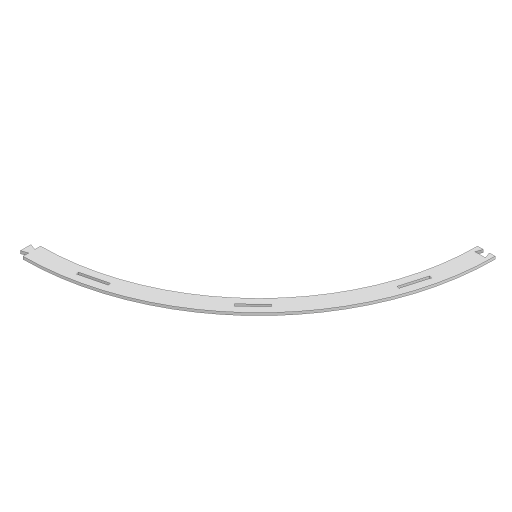
# Autodesk Inventor part: R50_CM_CIRCULO
Saved by Autodesk Inventor 2024.2 (Build 282272000, 272)
## iProperties
Created: 2024-10-01
Part Number: R50_CM_CIRCULO
Material: Generic
Document SubType Name: Modeling
Designer: jrcer
Density: 1 g/cm^3
Appearance: Default
Author: jrcer
Autodesk Inventor part; units mm, degrees
ref_plane "YZ Plane" through (0, 0, 0) normal (1, 0, 0) x (0, 1, 0)
ref_plane "XZ Plane" through (0, 0, 0) normal (0, 1, 0) x (-1, 0, 0)
ref_plane "XY Plane" through (0, 0, 0) normal (0, 0, 1) x (1, 0, 0)
sketch "Sketch1" plane through (0, 0, 0) normal (0, 1, 0) x (-1, 0, 0)
  circle A0 centre (0, 0) radius 250
  circle A1 centre (0, 0) radius 270
  line L0 (270, 0) -> (250, 0)
  line L1 (-270, 0) -> (-250, 0)
  line L2 (0, 0) -> (-250, 0) construction
  line L3 (0, 250) -> (0, 0) construction
  line L4 (0, 270) -> (0, 250)
  line L5 (-250, 0) -> (-270, 0)
  line L6 (-254, 7) -> (-266, 7)
  line L7 (-266, 7) -> (-263.4522, 0)
  line L8 (-254, 7) -> (-256.5478, 0)
  line L9 (-260, 0) -> (-260, 7) construction
  line L10 (-255.1125, 57.8859) -> (-246.8075, 86.7134)
  line L11 (-246.8075, 86.7134) -> (-243.7326, 85.8275)
  line L12 (-243.7326, 85.8275) -> (-252.0376, 57)
  line L13 (-252.0376, 57) -> (-255.1125, 57.8859)
  line L14 (-255.1125, 57.8859) -> (-243.7326, 85.8275) construction
  line L15 (-246.8075, 86.7134) -> (-252.0376, 57) construction
  circle A2 centre (0, 0) radius 260 construction
  line L16 (-7, -254) -> (0, -256.5478)
  line L17 (-7, -266) -> (0, -263.4522)
  line L18 (-7, -254) -> (-7, -266)
  line L19 (254, -7) -> (256.5478, 0)
  line L20 (266, -7) -> (263.4522, 0)
  line L21 (254, -7) -> (266, -7)
  line L22 (7, 254) -> (0, 256.5478)
  line L23 (7, 266) -> (0, 263.4522)
  line L24 (7, 254) -> (7, 266)
  line L25 (-249.8769, -77.4256) -> (-257.0983, -48.3078)
  line L26 (-246.771, -76.6553) -> (-249.8769, -77.4256)
  line L27 (-253.9924, -47.5375) -> (-246.771, -76.6553)
  line L28 (-257.0983, -48.3078) -> (-253.9924, -47.5375)
  line L29 (-177.6869, -191.991) -> (-198.4998, -170.3849)
  line L30 (-175.3822, -189.771) -> (-177.6869, -191.991)
  line L31 (-196.1951, -168.1649) -> (-175.3822, -189.771)
  line L32 (-198.4998, -170.3849) -> (-196.1951, -168.1649)
  line L33 (-57.8859, -255.1125) -> (-86.7134, -246.8075)
  line L34 (-57, -252.0376) -> (-57.8859, -255.1125)
  line L35 (-85.8275, -243.7326) -> (-57, -252.0376)
  line L36 (-86.7134, -246.8075) -> (-85.8275, -243.7326)
  line L37 (77.4256, -249.8769) -> (48.3078, -257.0983)
  line L38 (76.6553, -246.771) -> (77.4256, -249.8769)
  line L39 (47.5375, -253.9924) -> (76.6553, -246.771)
  line L40 (48.3078, -257.0983) -> (47.5375, -253.9924)
  line L41 (191.991, -177.6869) -> (170.3849, -198.4998)
  line L42 (189.771, -175.3822) -> (191.991, -177.6869)
  line L43 (168.1649, -196.1951) -> (189.771, -175.3822)
  line L44 (170.3849, -198.4998) -> (168.1649, -196.1951)
  line L45 (255.1125, -57.8859) -> (246.8075, -86.7134)
  line L46 (252.0376, -57) -> (255.1125, -57.8859)
  line L47 (243.7326, -85.8275) -> (252.0376, -57)
  line L48 (246.8075, -86.7134) -> (243.7326, -85.8275)
  line L49 (249.8769, 77.4256) -> (257.0983, 48.3078)
  line L50 (246.771, 76.6553) -> (249.8769, 77.4256)
  line L51 (253.9924, 47.5375) -> (246.771, 76.6553)
  line L52 (257.0983, 48.3078) -> (253.9924, 47.5375)
  line L53 (177.6869, 191.991) -> (198.4998, 170.3849)
  line L54 (175.3822, 189.771) -> (177.6869, 191.991)
  line L55 (196.1951, 168.1649) -> (175.3822, 189.771)
  line L56 (198.4998, 170.3849) -> (196.1951, 168.1649)
  line L57 (57.8859, 255.1125) -> (86.7134, 246.8075)
  line L58 (57, 252.0376) -> (57.8859, 255.1125)
  line L59 (85.8275, 243.7326) -> (57, 252.0376)
  line L60 (86.7134, 246.8075) -> (85.8275, 243.7326)
  line L61 (-77.4256, 249.8769) -> (-48.3078, 257.0983)
  line L62 (-76.6553, 246.771) -> (-77.4256, 249.8769)
  line L63 (-47.5375, 253.9924) -> (-76.6553, 246.771)
  line L64 (-48.3078, 257.0983) -> (-47.5375, 253.9924)
  line L65 (-191.991, 177.6869) -> (-170.3849, 198.4998)
  line L66 (-189.771, 175.3822) -> (-191.991, 177.6869)
  line L67 (-168.1649, 196.1951) -> (-189.771, 175.3822)
  line L68 (-170.3849, 198.4998) -> (-168.1649, 196.1951)
  point P0 (260, 0)
  point P1 (-260, 0)
  point P2 (-249.4226, 71.8567)
  point P3 (-49.7078, 255.2041)
  point P4 (-253.5751, 57.4429)
  point P5 (-245.2701, 86.2705)
  point P6 (-7, -260)
  point P7 (260, -7)
  point P8 (7, 260)
  point P9 (-248.3239, -77.0405)
  point P10 (-255.5453, -47.9226)
  point P11 (-176.5346, -190.881)
  point P12 (-197.3475, -169.2749)
  point P13 (-57.4429, -253.5751)
  point P14 (-86.2705, -245.2701)
  point P15 (77.0405, -248.3239)
  point P16 (47.9226, -255.5453)
  point P17 (190.881, -176.5346)
  point P18 (169.2749, -197.3475)
  point P19 (253.5751, -57.4429)
  point P20 (245.2701, -86.2705)
  point P21 (248.3239, 77.0405)
  point P22 (255.5453, 47.9226)
  point P23 (176.5346, 190.881)
  point P24 (197.3475, 169.2749)
  point P25 (57.4429, 253.5751)
  point P26 (86.2705, 245.2701)
  point P27 (-77.0405, 248.3239)
  point P28 (-47.9226, 255.5453)
  point P29 (-190.881, 176.5346)
  point P30 (-169.2749, 197.3475)
  point P31 (-256.5478, 0)
  point P32 (0, 256.5478)
  point P33 (0, 263.4522)
  dimension "d0" = 500
  dimension "d1" = 540
  dimension "d4" = 90
  dimension "d5" = 7
  dimension "d6" = 70
  dimension "d8" = 12
  dimension "d13" = 3.2
  dimension "d14" = 30
  dimension "d15" = 50
  dimension "d20" = 520
  dimension "d23" = 360
  dimension "d27" = 360
  constraints: 138 end point, 11 point on circle, 8 midpoint, 3 centre point, 3 coincident, 3 parallel, 2 horizontal, 2 horizontal alignment, 2 perpendicular, 2 point on line, 2 vertical, 1 collinear, 1 equal length, 154 other
  measures "d0" diameter of A0
  measures "d1" diameter of A1
  measures "d4" angle of L2 L3
  measures "d5" distance between parallel lines of L6 L5
  measures "d6" angle of L7 L6
  measures "d8" distance of L6.start L6.end
  measures "d13" distance of L10.end L11.end
  measures "d14" distance of L11.end L12.end
  measures "d15" vertical distance of L12.end L6.start
  measures "d20" diameter of A2
extrude "Extrusion1" add sketch "Sketch1" along normal blind 3 contours A0 L1 L8 L6 L7 A1 L4 | L4 L23 L24 L22
body "Solid1"
